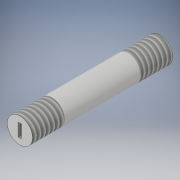
# Autodesk Inventor part: Pedal Axle
Saved by Autodesk Inventor 2019 (Build 230136000, 136)
## iProperties
Created: 2020-06-01
Part Number: Pedal Axle
Material: Generic
Document SubType Name: Modeling
Designer: 18186
Density: 1 g/cm^3
Appearance: Default
Author: 18186
Autodesk Inventor part; units mm, degrees
ref_plane "YZ Plane" through (0, 0, 0) normal (1, 0, 0) x (0, 1, 0)
ref_plane "XZ Plane" through (0, 0, 0) normal (0, 1, 0) x (-1, 0, 0)
ref_plane "XY Plane" through (0, 0, 0) normal (0, 0, 1) x (1, 0, 0)
sketch "Sketch1" plane through (0, 0, 0) normal (0, 0, 1) x (1, 0, 0)
  circle A0 centre (0, 0) radius 5
  dimension "d0" = 10
  constraints: 1 centre point, 1 coincident
  measures "d0" diameter of A0
extrude "Extrusion1" add sketch "Sketch1" along normal blind 12.7
sketch "Sketch2" plane through (0, 0, 12.7) normal (0, 0, 1) x (1, 0, 0)
  point P0 (0, 0)
thread "Thread1" size "7/16-14 UNC" class "2A" standard "ANSI Unified Screw Threads" length 12.7
ref_plane "Work Plane1" through (0, 0, 42.78) normal (0, 0, 1) x (1, 0, 0)
sketch "Sketch3" plane through (0, 0, 42.78) normal (0, 0, 1) x (1, 0, 0)
  circle A0 centre (0, 0) radius 5 projected
extrude "Extrusion2" add sketch "Sketch3" along normal blind 12.7
thread "Thread2" size "7/16-14 UNC" class "2A" standard "ANSI Unified Screw Threads" length 12.7
sketch "Sketch4" plane through (0, 0, 42.78) normal (0, 0, -1) x (-1, 0, 0)
  circle A0 centre (0, 0) radius 5
  constraints: 1 centre point, 1 coincident
extrude "Extrusion3" add sketch "Sketch4" along normal blind 30.08
sketch "Sketch5" plane through (0, 0, 55.48) normal (0, 0, 1) x (1, 0, 0)
  line L0 (-0.635, 2.54) -> (0.635, 2.54)
  line L1 (0.635, 2.54) -> (0.635, -2.54)
  line L2 (0.635, -2.54) -> (-0.635, -2.54)
  line L3 (-0.635, -2.54) -> (-0.635, 2.54)
  line L4 (-0.635, 2.54) -> (0.635, -2.54) construction
  line L5 (0.635, 2.54) -> (-0.635, -2.54) construction
  point P0 (0, 0)
  dimension "d15" = 1.27
  dimension "d16" = 5.08
  constraints: 12 end point, 2 midpoint, 2 parallel, 1 horizontal, 1 perpendicular
  measures "d15" distance of L1.end L2.end
  measures "d16" distance of L0.end L1.end
extrude "Extrusion4" cut sketch "Sketch5" against normal through all
body "Solid1"
